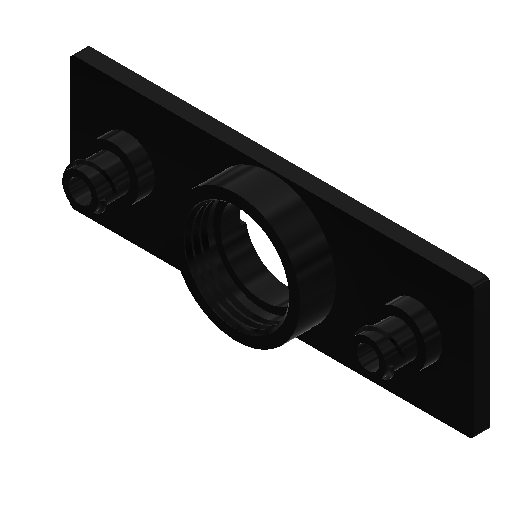
# Autodesk Inventor part: PRT - 9301 - MFLEAFCHIP - V04 - B
Saved by Autodesk Inventor 2025.3 (Build 293356000, 356)
## iProperties
Part Number: PRT - 9301 - MFLEAFCHIP - V04 - B
Material: Generic
Description: Leaf chamber chip B (luer inlet -> chamber -> luer outlet), print in black resin
Document SubType Name: Modeling
Designer: benir
Appearance: Low Gloss - Black
Author: benir
Autodesk Inventor part; units mm, degrees
ref_plane "z = -cs_recess" through (0, 0, -0.25) normal (0, 0, 1) x (1, 0, 0)
sketch "slab sketch" plane through (0, 0, -0.25) normal (0, 0, 1) x (1, 0, 0)
  line L0 (-38, -12.5) -> (38, -12.5)
  line L1 (38, -12.5) -> (38, 12.5)
  line L2 (38, 12.5) -> (-38, 12.5)
  line L3 (-38, 12.5) -> (-38, -12.5)
  line L4 (0, -17.5) -> (0, 17.5) projected
  line L5 (-53.2, 0) -> (53.2, 0) projected
  dimension "d1" = 76
  dimension "d2" = 25
  constraints: 8 end point, 2 parallel, 1 horizontal, 1 perpendicular, 2 other
  measures "d1" distance of L0.start L0.end
  measures "d2" distance of L2.end L0.start
extrude "slab" add sketch "slab sketch" along normal blind 3.25
fillet "slab corners" radius 1 4 edges at (-38, -12.5, 1.375) (-38, 12.5, 1.375) (38, 12.5, 1.375) (38, -12.5, 1.375)
sketch "glue band sketch" plane through (0, 0, 0) normal (0, 0, 1) x (1, 0, 0)
  line L0 (-130.25, -13.5) -> (130.25, -13.5)
  line L1 (130.25, -13.5) -> (130.25, 13.5)
  line L2 (130.25, 13.5) -> (-130.25, 13.5)
  line L3 (-130.25, 13.5) -> (-130.25, -13.5)
  line L4 (0, -18.9) -> (0, 18.9) projected
  line L5 (-182.35, 0) -> (182.35, 0) projected
  dimension "d6" = 260.5
  dimension "d7" = 27
  constraints: 8 end point, 2 parallel, 1 horizontal, 1 perpendicular, 2 other
  measures "d6" distance of L0.start L0.end
  measures "d7" distance of L2.end L0.start
extrude "glue band (bottom coverslip)" cut sketch "glue band sketch" against normal blind 0.75
ref_plane "z = base_t" through (0, 0, 3) normal (0, 0, 1) x (1, 0, 0)
sketch "chamber boss sketch" plane through (0, 0, 3) normal (0, 0, 1) x (1, 0, 0)
  circle A0 centre (0, 0) radius 12
  dimension "d11" = 24
  constraints: 1 centre point
  measures "d11" diameter of A0
extrude "chamber boss" add sketch "chamber boss sketch" along normal blind 6.7
sketch "inlet luer foot sketch" plane through (0, 0, 3) normal (0, 0, 1) x (1, 0, 0)
  circle A0 centre (27, 0) radius 5
  line L0 (-6.4, 0) -> (38.4, 0) projected
  point P0 (0, 0)
  dimension "d14" = 27
  dimension "d15" = 10
  constraints: 1 centre point, 1 point on line
  measures "d14" distance of point (0, 0) A0.centre
  measures "d15" diameter of A0
extrude "inlet luer foot" add sketch "inlet luer foot sketch" along normal blind 3
sketch "inlet luer hub sketch" plane through (0, 0, 3) normal (0, 0, 1) x (1, 0, 0)
  circle A0 centre (27, 0) radius 3.365
  line L0 (-6.073, 0) -> (36.438, 0) projected
  point P0 (0, 0)
  dimension "d18" = 27
  dimension "d19" = 6.73
  constraints: 1 centre point, 1 point on line
  measures "d18" distance of point (0, 0) A0.centre
  measures "d19" diameter of A0
extrude "inlet luer hub" add sketch "inlet luer hub sketch" along normal blind 9
ref_plane "x = in_x" through (27, 0, 0) normal (1, 0, 0) x (0, 1, 0)
sketch "inlet luer lug profile" plane through (0, 0, 0) normal (0, 1, 0) x (-1, 0, 0)
  line L0 (-30.265, 8.25) -> (-30.915, 8.55)
  line L1 (-30.915, 8.55) -> (-30.915, 8.9)
  line L2 (-30.915, 8.9) -> (-30.265, 9.2)
  line L3 (-30.265, 9.2) -> (-30.265, 8.25)
  point P0 (0, 0)
  dimension "d23" = 8.25
  dimension "d24" = 30.265
  dimension "d25" = 8.55
  dimension "d26" = 30.915
  dimension "d27" = 8.9
  dimension "d28" = 30.915
  dimension "d29" = 9.2
  dimension "d30" = 30.265
  constraints: 8 end point
  measures "d23" vertical distance of point (0, 0) L0.start
  measures "d24" horizontal distance of point (0, 0) L0.start
  measures "d25" vertical distance of point (0, 0) L0.end
  measures "d26" horizontal distance of point (0, 0) L0.end
  measures "d27" vertical distance of point (0, 0) L1.end
  measures "d28" horizontal distance of point (0, 0) L1.end
  measures "d29" vertical distance of point (0, 0) L2.end
  measures "d30" horizontal distance of point (0, 0) L2.end
coil "inlet luer lug (RH, lead luer_lead)" sketch "inlet luer lug profile" operation add axis through (27, 0, 0) along (0, 0, 1) pitch 5 turns 0.5 hand right
pattern_circular "inlet luer lugs x2" count 2 over 360 about axis through (27, 0, 0) along (0, 0, 1) of "inlet luer lug (RH, lead luer_lead)"
sketch "outlet luer foot sketch" plane through (0, 0, 3) normal (0, 0, 1) x (1, 0, 0)
  circle A0 centre (-27, 0) radius 5
  line L0 (-38.4, 0) -> (6.4, 0) projected
  point P0 (0, 0)
  dimension "d42" = 27
  dimension "d43" = 10
  constraints: 1 centre point, 1 point on line
  measures "d42" distance of point (0, 0) A0.centre
  measures "d43" diameter of A0
extrude "outlet luer foot" add sketch "outlet luer foot sketch" along normal blind 3
sketch "outlet luer hub sketch" plane through (0, 0, 3) normal (0, 0, 1) x (1, 0, 0)
  circle A0 centre (-27, 0) radius 3.365
  line L0 (-36.438, 0) -> (6.073, 0) projected
  point P0 (0, 0)
  dimension "d46" = 27
  dimension "d47" = 6.73
  constraints: 1 centre point, 1 point on line
  measures "d46" distance of point (0, 0) A0.centre
  measures "d47" diameter of A0
extrude "outlet luer hub" add sketch "outlet luer hub sketch" along normal blind 9
ref_plane "x = -out_x" through (-27, 0, 0) normal (1, 0, 0) x (0, 1, 0)
sketch "outlet luer lug profile" plane through (0, 0, 0) normal (0, 1, 0) x (-1, 0, 0)
  line L0 (23.735, 8.25) -> (23.085, 8.55)
  line L1 (23.085, 8.55) -> (23.085, 8.9)
  line L2 (23.085, 8.9) -> (23.735, 9.2)
  line L3 (23.735, 9.2) -> (23.735, 8.25)
  point P0 (0, 0)
  dimension "d51" = 8.25
  dimension "d52" = 23.735
  dimension "d53" = 8.55
  dimension "d54" = 23.085
  dimension "d55" = 8.9
  dimension "d56" = 23.085
  dimension "d57" = 9.2
  dimension "d58" = 23.735
  constraints: 8 end point
  measures "d51" vertical distance of point (0, 0) L0.start
  measures "d52" horizontal distance of point (0, 0) L0.start
  measures "d53" vertical distance of point (0, 0) L0.end
  measures "d54" horizontal distance of point (0, 0) L0.end
  measures "d55" vertical distance of point (0, 0) L1.end
  measures "d56" horizontal distance of point (0, 0) L1.end
  measures "d57" vertical distance of point (0, 0) L2.end
  measures "d58" horizontal distance of point (0, 0) L2.end
coil "outlet luer lug (RH, lead luer_lead)" sketch "outlet luer lug profile" operation add axis through (-27, 0, 0) along (0, 0, 1) pitch 5 turns 0.5 hand right
pattern_circular "outlet luer lugs x2" count 2 over 360 about axis through (-27, 0, 0) along (0, 0, 1) of "outlet luer lug (RH, lead luer_lead)"
sketch "well sketch" plane through (0, 0, 0) normal (0, 0, 1) x (1, 0, 0)
  circle A0 centre (0, 0) radius 7.15
  dimension "d70" = 14.3
  constraints: 1 centre point
  measures "d70" diameter of A0
extrude "chamber well" cut sketch "well sketch" along normal blind 4.7
ref_plane "z = ledge_z" through (0, 0, 4.7) normal (0, 0, 1) x (1, 0, 0)
sketch "thread bore sketch" plane through (0, 0, 4.7) normal (0, 0, 1) x (1, 0, 0)
  circle A0 centre (0, 0) radius 9.338125
  dimension "d74" = 18.67625
  constraints: 1 centre point
  measures "d74" diameter of A0
extrude "thread bore" cut sketch "thread bore sketch" along normal blind 6
chamfer "thread lead-in" distance 0.6 angle 45 1 edges at (-9.3381, 0, 9.7)
chamfer "O-ring lead-in" distance 0.6 angle 45 1 edges at (-7.15, 0, 4.7)
sketch "internal thread groove profile" plane through (0, 0, 0) normal (0, 1, 0) x (-1, 0, 0)
  line L0 (-9.238125, 5) -> (-10.15, 5.526471)
  line L1 (-10.15, 5.526471) -> (-10.15, 5.713971)
  line L2 (-10.15, 5.713971) -> (-9.238125, 6.240442)
  line L3 (-9.238125, 6.240442) -> (-9.238125, 5)
  point P0 (0, 0)
  dimension "d83" = 5
  dimension "d84" = 9.23813
  dimension "d85" = 5.52647
  dimension "d86" = 10.15
  dimension "d87" = 5.71397
  dimension "d88" = 10.15
  dimension "d89" = 6.24044
  dimension "d90" = 9.23813
  constraints: 8 end point
  measures "d83" vertical distance of point (0, 0) L0.start
  measures "d84" horizontal distance of point (0, 0) L0.start
  measures "d85" vertical distance of point (0, 0) L0.end
  measures "d86" horizontal distance of point (0, 0) L0.end
  measures "d87" vertical distance of point (0, 0) L1.end
  measures "d88" horizontal distance of point (0, 0) L1.end
  measures "d89" vertical distance of point (0, 0) L2.end
  measures "d90" horizontal distance of point (0, 0) L2.end
coil "M20x1.5 internal thread (coil cut, RH)" sketch "internal thread groove profile" operation cut axis through (0, 0, -10) along (0, 0, 1) pitch 1.5 turns 3.719853 hand right
ref_plane "z = luer_top" through (0, 0, 12) normal (0, 0, 1) x (1, 0, 0)
sketch "inlet luer bore sketch" plane through (0, 0, 12) normal (0, 0, 1) x (1, 0, 0)
  circle A0 centre (27, 0) radius 2.145
  line L0 (-5.829, 0) -> (34.974, 0) projected
  point P0 (0, 0)
  dimension "d100" = 27
  dimension "d101" = 4.29
  constraints: 1 centre point, 1 point on line
  measures "d100" distance of point (0, 0) A0.centre
  measures "d101" diameter of A0
sketch "inlet luer bore sketch outline for inlet luer taper bore (6 %)" plane through (0, 0, 12) normal (0, 0, 1) x (1, 0, 0)
  circle A0 centre (27, 0) radius 2.145
extrude "inlet luer taper bore (6 %)" cut sketch "inlet luer bore sketch outline for inlet luer taper bore (6 %)" against normal blind 8 draft -1.71836
sketch "outlet luer bore sketch" plane through (0, 0, 12) normal (0, 0, 1) x (1, 0, 0)
  circle A0 centre (-27, 0) radius 2.145
  line L0 (-34.974, 0) -> (5.829, 0) projected
  point P0 (0, 0)
  dimension "d104" = 27
  dimension "d105" = 4.29
  constraints: 1 centre point, 1 point on line
  measures "d104" distance of point (0, 0) A0.centre
  measures "d105" diameter of A0
sketch "outlet luer bore sketch outline for outlet luer taper bore (6 %)" plane through (0, 0, 12) normal (0, 0, 1) x (1, 0, 0)
  circle A0 centre (-27, 0) radius 2.145
extrude "outlet luer taper bore (6 %)" cut sketch "outlet luer bore sketch outline for outlet luer taper bore (6 %)" against normal blind 8 draft -1.71836
ref_plane "z = ch_floor" through (0, 0, 0) normal (0, 0, 1) x (1, 0, 0)
sketch "channel sketch" plane through (0, 0, 0) normal (0, 0, 1) x (1, 0, 0)
  line L0 (3.575, -1.5) -> (27, -1.5)
  line L1 (27, -1.5) -> (27, 1.5)
  line L2 (27, 1.5) -> (3.575, 1.5)
  line L3 (3.575, 1.5) -> (3.575, -1.5)
  line L4 (-37.8, 0) -> (37.8, 0) projected
  line L5 (-27, -1.5) -> (-3.575, -1.5)
  line L6 (-3.575, -1.5) -> (-3.575, 1.5)
  line L7 (-3.575, 1.5) -> (-27, 1.5)
  line L8 (-27, 1.5) -> (-27, -1.5)
  point P0 (0, 0)
  dimension "d109" = 3
  dimension "d110" = 3.575
  dimension "d111" = 27
  dimension "d112" = 3
  dimension "d113" = 27
  dimension "d114" = 3.575
  constraints: 16 end point, 4 parallel, 2 horizontal, 2 perpendicular, 2 other
  measures "d109" distance of L2.end L0.start
  measures "d110" horizontal distance of point (0, 0) L2.end
  measures "d111" horizontal distance of point (0, 0) L0.end
  measures "d112" distance of L7.end L5.start
  measures "d113" horizontal distance of point (0, 0) L7.end
  measures "d114" horizontal distance of point (0, 0) L5.end
extrude "channels" cut sketch "channel sketch" along normal blind 1
sketch "inlet via sketch" plane through (0, 0, 0) normal (0, 0, 1) x (1, 0, 0)
  circle A0 centre (27, 0) radius 1
  line L0 (-5.6, 0) -> (33.6, 0) projected
  point P0 (0, 0)
  dimension "d117" = 27
  dimension "d118" = 2
  constraints: 1 centre point, 1 point on line
  measures "d117" distance of point (0, 0) A0.centre
  measures "d118" diameter of A0
extrude "inlet via" cut sketch "inlet via sketch" along normal blind 4.3
sketch "outlet via sketch" plane through (0, 0, 0) normal (0, 0, 1) x (1, 0, 0)
  circle A0 centre (-27, 0) radius 1
  line L0 (-33.6, 0) -> (5.6, 0) projected
  point P0 (0, 0)
  dimension "d121" = 27
  dimension "d122" = 2
  constraints: 1 centre point, 1 point on line
  measures "d121" distance of point (0, 0) A0.centre
  measures "d122" diameter of A0
extrude "outlet via" cut sketch "outlet via sketch" along normal blind 4.3
sketch "Sketch18" plane through (0, 0, 4.7) normal (0, 0, 1) x (1, 0, 0)
  circle A0 centre (0, 0) radius 7.15 projected
  circle A1 centre (0, 0) radius 8
  dimension "d125" = 16
  constraints: 1 centre point, 1 coincident
  measures "d125" diameter of A1
extrude "Extrusion15" cut sketch "Sketch18" against normal through all
equation "\"d2\" = chip_w"
equation "\"d3\" = base_t + cs_recess"
equation "\"d5\" = corner_r"
equation "\"d11\" = boss_d"
equation "\"d12\" = boss_top - base_t"
equation "\"d14\" = in_x"
equation "\"d15\" = luer_foot_d"
equation "\"d16\" = -luer_free + luer_top - base_t"
equation "\"d18\" = in_x"
equation "\"d19\" = luer_hub_d"
equation "\"d20\" = luer_top - base_t"
equation "\"d23\" = lug_zc - 0.5 * luer_lug_base"
equation "\"d24\" = in_x + lug_r_in"
equation "\"d25\" = lug_zc - 0.5 * luer_lug_crest"
equation "\"d26\" = in_x + 0.5 * luer_lug_d"
equation "\"d27\" = lug_zc + 0.5 * luer_lug_crest"
equation "\"d28\" = in_x + 0.5 * luer_lug_d"
equation "\"d29\" = lug_zc + 0.5 * luer_lug_base"
equation "\"d30\" = in_x + lug_r_in"
equation "\"d31\" = luer_lead"
equation "\"d33\" = luer_lug_rev"
equation "\"d42\" = out_x"
equation "\"d43\" = luer_foot_d"
equation "\"d44\" = -luer_free + luer_top - base_t"
equation "\"d46\" = out_x"
equation "\"d47\" = luer_hub_d"
equation "\"d48\" = luer_top - base_t"
equation "\"d51\" = lug_zc - 0.5 * luer_lug_base"
equation "\"d52\" = -lug_r_in + out_x"
equation "\"d53\" = lug_zc - 0.5 * luer_lug_crest"
equation "\"d54\" = -0.5 * luer_lug_d + out_x"
equation "\"d55\" = lug_zc + 0.5 * luer_lug_crest"
equation "\"d56\" = -0.5 * luer_lug_d + out_x"
equation "\"d57\" = lug_zc + 0.5 * luer_lug_base"
equation "\"d58\" = -lug_r_in + out_x"
equation "\"d59\" = luer_lead"
equation "\"d61\" = luer_lug_rev"
equation "\"d70\" = well_d"
equation "\"d71\" = ledge_z"
equation "\"d74\" = th_bore_d"
equation "\"d77\" = th_chamfer"
equation "\"d78\" = th_chamfer"
equation "\"d80\" = well_chamfer"
equation "\"d81\" = well_chamfer"
equation "\"d83\" = ti_zc - 0.5 * ti_w_in"
equation "\"d84\" = ti_r_in"
equation "\"d85\" = ti_zc - 0.5 * ti_w_root"
equation "\"d86\" = 0.5 * th_root_d"
equation "\"d87\" = ti_zc + 0.5 * ti_w_root"
equation "\"d88\" = 0.5 * th_root_d"
equation "\"d89\" = ti_zc + 0.5 * ti_w_in"
equation "\"d90\" = ti_r_in"
equation "\"d91\" = th_p"
equation "\"d92\" = ti_height"
equation "\"d100\" = in_x"
equation "\"d101\" = luer_open_d"
equation "\"d102\" = luer_depth"
equation "\"d103\" = -luer_taper_deg"
equation "\"d104\" = out_x"
equation "\"d105\" = luer_open_d"
equation "\"d106\" = luer_depth"
equation "\"d107\" = -luer_taper_deg"
equation "\"d109\" = ch_w"
equation "\"d110\" = 0.25 * well_d"
equation "\"d111\" = in_x"
equation "\"d112\" = ch_w"
equation "\"d113\" = out_x"
equation "\"d114\" = 0.25 * well_d"
equation "\"d115\" = ch_h"
equation "\"d117\" = in_x"
equation "\"d118\" = via_d"
equation "\"d121\" = out_x"
equation "\"d122\" = via_d"
equation "\"cs_recess\" = 0.25"
equation "\"d0\" = -cs_recess"
equation "\"chip_l\" = 75"
equation "\"chip_w\" = 25"
equation "\"base_t\" = 3"
equation "\"corner_r\" = 1"
equation "\"cs_gap\" = 0.25"
equation "\"d10\" = base_t"
equation "\"boss_d\" = 24"
equation "\"chamber_h\" = 1.5"
equation "\"stub_len\" = 3.2"
equation "\"ledge_z\" = chamber_h + stub_len"
equation "\"th_len\" = 5"
equation "\"boss_top\" = ledge_z + th_len"
equation "\"in_x\" = 27"
equation "\"luer_foot_d\" = 10"
equation "\"luer_top\" = 12"
equation "\"luer_free\" = 6"
equation "\"luer_hub_d\" = 6.73"
equation "\"d22\" = in_x"
equation "\"luer_lug_gap\" = 0.3"
equation "\"luer_lug_base\" = 0.95"
equation "\"luer_lug_rev\" = 0.5"
equation "\"luer_lead\" = 5"
equation "\"luer_lug_d\" = 7.83"
equation "\"luer_lug_crest\" = 0.35"
equation "\"out_x\" = 27"
equation "\"d50\" = -out_x"
equation "\"well_d\" = 14.3"
equation "\"d73\" = ledge_z"
equation "\"th_p\" = 1.5"
equation "\"th_clear\" = 0.15"
equation "\"th_bore_d\" = -1.0825 * th_p + th_d + 2 * th_clear"
equation "\"th_chamfer\" = 0.6"
equation "\"well_chamfer\" = 0.6"
equation "\"th_start\" = 0.3"
equation "\"ti_w_root\" = 0.125 * th_p"
equation "\"th_root_d\" = th_d + 2 * th_clear"
equation "\"ti_w_in\" = ti_w_root + 0.57735 * th_root_d - 1.1547 * ti_r_in"
equation "\"ti_zc\" = th_start + ledge_z + 0.5 * ti_w_in"
equation "\"ti_height\" = th_p + boss_top - ti_zc"
equation "\"d99\" = luer_top"
equation "\"luer_open_d\" = 4.29"
equation "\"luer_depth\" = 8"
equation "\"luer_taper_deg\" = 1.71836deg"
equation "\"ch_floor\" = 0"
equation "\"ch_w\" = 3"
equation "\"ch_h\" = 1"
equation "\"via_d\" = 2"
equation "\"luer_bot_z\" = luer_top - luer_depth"
equation "\"th_d\" = 20"
equation "\"ti_r_in\" = 9.238125"
equation "\"lug_zc\" = 8.725"
equation "\"lug_r_in\" = 3.265"
body "Solid1"
